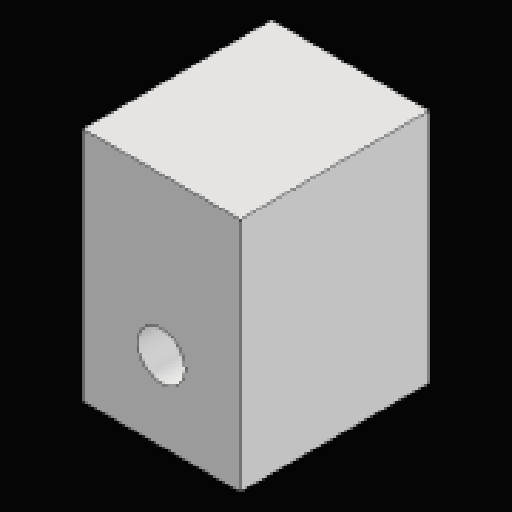
# Autodesk Inventor part: Rack
Saved by Autodesk Inventor 2023.2 (Build 272271030, 271C)
## iProperties
Created: 2023-11-11
Part Number: Rack
Material: Generic
Document SubType Name: Modeling
Designer: robpl
Density: 1 g/cm^3
Appearance: Default
Author: robpl
Autodesk Inventor part; units mm, degrees
ref_plane "YZ Plane" through (0, 0, 0) normal (1, 0, 0) x (0, 1, 0)
ref_plane "XZ Plane" through (0, 0, 0) normal (0, 1, 0) x (-1, 0, 0)
ref_plane "XY Plane" through (0, 0, 0) normal (0, 0, 1) x (1, 0, 0)
sketch "Sketch1" plane through (0, 0, 0) normal (0, 0, 1) x (1, 0, 0)
  line L0 (0, 0) -> (10, 0)
  line L1 (10, 0) -> (10, 10)
  line L2 (10, 10) -> (0, 10)
  line L3 (0, 10) -> (0, 0)
  line L4 (0, 0) -> (-5, 0)
  line L5 (-5, 0) -> (-5, 7)
  line L6 (-5, 7) -> (0, 7)
  line L7 (0, 7) -> (0, 0)
  point P0 (0, 7)
  dimension "d0" = 10
  dimension "d1" = 10
  dimension "d8" = 5
  dimension "d9" = 7
  constraints: 16 end point, 4 parallel, 2 horizontal, 2 perpendicular
  measures "d0" distance of L2.end L1.end
  measures "d1" distance of L1.end L0.end
  measures "d8" distance of L5.end L6.end
  measures "d9" distance of L4.end L5.end
extrude "Extrusion1" add sketch "Sketch1" along normal blind 12
sketch "Sketch2" plane through (0, 0, 12) normal (0, 0, 1) x (1, 0, 0)
  circle A0 centre (5, 5) radius 1.5
  line L0 (10, 0) -> (10, 10) projected
  line L1 (10, 10) -> (0, 10) projected
  line L2 (0, 10) -> (0, 7) projected
  line L3 (0, 7) -> (-5, 7) projected
  line L4 (-5, 7) -> (-5, 0) projected
  line L5 (-5, 0) -> (10, 0) projected
  point P0 (0, 0)
  point P1 (5, 0)
  dimension "d4" = 3
  constraints: 1 centre point, 1 vertical alignment
  measures "d4" diameter of A0
extrude "Extrusion2" cut sketch "Sketch2" against normal through all contours A0
body "Solid1"
